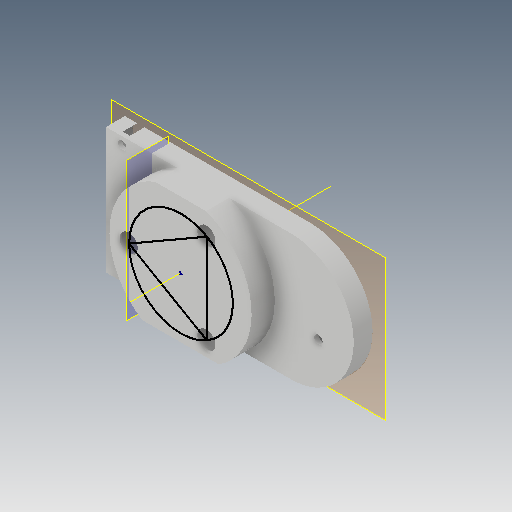
# Autodesk Inventor part: 03_Insert_Chip_solid
Saved by Autodesk Inventor 2019 (Build 230136000, 136)
## iProperties
Created: 2019-06-11
Part Number: 03_Insert_Chip_solid
Material: Generic
Document SubType Name: Modeling
Designer: diederichbenedict
Density: 1 g/cm^3
Appearance: Default
Author: diederichbenedict
Autodesk Inventor part; units mm, degrees
ref_plane "YZ Plane" through (0, 0, 0) normal (1, 0, 0) x (0, 1, 0)
ref_plane "XZ Plane" through (0, 0, 0) normal (0, 1, 0) x (-1, 0, 0)
ref_plane "XY Plane" through (0, 0, 0) normal (0, 0, 1) x (1, 0, 0)
ref_plane "Work Plane1" through (-1.2111, 0.775, 9.6) normal (0, 0, 1) x (0, -1, 0)
sketch "Sketch1" plane through (-1.2111, 0.775, 9.6) normal (0, 0, 1) x (0, -1, 0)
  circle A0 centre (3.575, 28.5389) radius 1.75 construction
  circle A1 centre (-13.125, -18.1803) radius 2 construction
  arc A2 (15.225, -15.8355) -> (15.225, -18.7868) centre (13.875, -17.3111) ccw construction
  line L0 (15.225, -15.8355) -> (15.225, 22.2111) construction
  arc A3 (15.225, 22.2111) -> (-15.225, 22.2111) centre (0, 21.8802) ccw construction
  line L1 (-15.225, 22.2111) -> (-15.225, -22.2111) construction
  line L2 (-15.225, -22.2111) -> (15.225, -22.2111) construction
  line L3 (15.225, -22.2111) -> (15.225, -18.7868) construction
  arc A4 (15.025, 22.209) -> (-15.025, 22.209) centre (0, 21.8802) ccw
  line L4 (15.025, 22.209) -> (15.025, -15.4356)
  arc A5 (15.025, -15.4356) -> (15.025, -19.1866) centre (13.875, -17.3111) ccw
  line L5 (15.025, -19.1866) -> (15.025, -22.0111)
  line L6 (15.025, -22.0111) -> (-14.956, -22.0111)
  arc A6 (-15.025, -18.8048) -> (-15.025, -17.5558) centre (-13.125, -18.1803) ccw construction
  circle A7 centre (3.575, 28.5389) radius 2.25
  arc A8 (-14.9598, -19.0514) -> (-14.9748, -17.3415) centre (-13.125, -18.1803) ccw
  line L7 (-14.956, -22.0111) -> (-14.9598, -19.0514)
  line L8 (-14.9748, -17.3415) -> (-15.025, 22.209)
  point P0 (0.775, 1.2111)
  dimension "d0" = 0.2
  dimension "d1" = 0.5
  constraints: 10 end point, 10 point on circle, 5 centre point, 1 coincident, 1 concentric, 1 parallel, 4 other
  measures "d0" radial gap between concentric circles of A3 A4
  measures "d1" radial gap between concentric circles of A0 A7
ref_plane "Work Plane2" through (21, -90, 18.7376) normal (0, 0, 1) x (1, 0, 0)
extrude "Extrusion1" add sketch "Sketch1" along normal blind 10
sketch "Sketch2" plane through (-16.6468, -14.25, 19.6) normal (0, 0, 1) x (1, 0, 0)
  circle A0 centre (16.6468, 14.25) radius 12.3406
  line L0 (4.3062, 14.25) -> (22.8171, 24.9373)
  line L1 (22.8171, 24.9373) -> (22.8171, 3.5627)
  line L2 (22.8171, 3.5627) -> (4.3062, 14.25)
  constraints: 6 end point, 2 coincident, 1 horizontal alignment, 9 other
ref_plane "Work Plane3" through (-12.3406, 0, 19.6) normal (-1, 0, 0) x (0, 0, 1)
sketch "Sketch3" plane through (-12.3406, 0, 19.6) normal (-1, 0, 0) x (0, 0, 1)
  line L0 (-0.8319, 0) -> (-10, 0)
  line L1 (-10, 15.8) -> (-10, -14.25) projected
  circle A0 centre (-1.4284, 0) radius 2.6
  line L2 (1.1716, 0) -> (-4.0284, 0)
  point P0 (-19.6, 0)
  dimension "d4" = 5.2
  constraints: 4 end point, 3 point on line, 2 point on circle, 1 centre point, 1 horizontal
  measures "d4" diameter of A0
revolve "Revolution1" cut sketch "Sketch3" angle 360 about axis through (-12.3406, 0, 18.7681) along (0, 0, -1) picked at (-2.9377, -0.2074) contours L2 A0 L0
pattern_circular "Circular Pattern1" count 3 over 360 about axis through (0, 0, 19.6) along (0, 0, 1) of "Revolution1"
ref_plane "Work Plane4" through (25.5777, -4.55, 13.1) normal (0, 0, 1) x (1, 0, 0)
sketch "Sketch5" plane through (-1.2111, 0.775, 19.6) normal (0, 0, 1) x (1, 0, 0)
  circle A0 centre (1.2111, -0.775) radius 16.9061
  circle A1 centre (7.3815, 9.9123) radius 2.1725 projected
  circle A2 centre (7.3815, -11.4623) radius 2.1725 projected
  circle A3 centre (-11.1295, -0.775) radius 2.1725 projected
  circle A4 centre (28.5389, -3.575) radius 2.25 projected
  arc A5 (22.209, -15.025) -> (22.209, 15.025) centre (21.8802, 0) ccw projected
  line L0 (22.209, 15.025) -> (-17.3415, 14.9748) projected
  arc A6 (-19.0514, 14.9598) -> (-17.3415, 14.9748) centre (-18.1803, 13.125) ccw projected
  line L1 (-19.0514, 14.9598) -> (-22.0111, 14.956) projected
  line L2 (-22.0111, 14.956) -> (-22.0111, -15.025) projected
  line L3 (-22.0111, -15.025) -> (-19.1866, -15.025) projected
  arc A7 (-15.4356, -15.025) -> (-19.1866, -15.025) centre (-17.3111, -13.875) ccw projected
  line L4 (-15.4356, -15.025) -> (22.209, -15.025) projected
  line L5 (22.209, 15.025) -> (-17.3415, 14.9748) projected
  line L6 (-15.4356, -15.025) -> (22.209, -15.025) projected
  point P0 (7.2754, 15.006)
  point P1 (-4.8932, 14.9906)
  point P2 (-7.8858, -15.025)
  point P3 (10.3081, -15.025)
  constraints: 4 point on circle, 4 point on line, 1 centre point, 1 coincident
extrude "Extrusion3" cut sketch "Sketch5" against normal up to surface (6.5 mm away) contours A0 L0 A5 L4 | A0 L4 A7 L3 L2 L1 A6 L0
sketch "Sketch6" plane through (-1.2111, 0.775, 13.1) normal (0, 0, 1) x (1, 0, 0)
  circle A0 centre (28.5389, -3.575) radius 2.25 projected
  arc A1 (22.209, -15.025) -> (22.209, 15.025) centre (21.8802, 0) ccw projected
  line L0 (7.2754, 15.006) -> (22.209, 15.025) projected
  arc A2 (10.3081, -15.025) -> (7.2754, 15.006) centre (1.2111, -0.775) ccw projected
  line L1 (22.209, -15.025) -> (10.3081, -15.025) projected
  arc A3 (-19.0514, 14.9598) -> (-17.3415, 14.9748) centre (-18.1803, 13.125) ccw projected
  line L2 (-22.0111, 14.956) -> (-19.0514, 14.9598) projected
  line L3 (-22.0111, -15.025) -> (-22.0111, 14.956) projected
  line L4 (-19.1866, -15.025) -> (-22.0111, -15.025) projected
  arc A4 (-15.4356, -15.025) -> (-19.1866, -15.025) centre (-17.3111, -13.875) ccw projected
  line L5 (-7.8858, -15.025) -> (-15.4356, -15.025) projected
  arc A5 (-4.8932, 14.9906) -> (-7.8858, -15.025) centre (1.2111, -0.775) ccw projected
  line L6 (-17.3415, 14.9748) -> (-4.8932, 14.9906) projected
  circle A6 centre (-18.1803, 13.125) radius 1
  circle A7 centre (-17.3111, -13.875) radius 1
  circle A8 centre (28.5389, -3.575) radius 1
  arc A9 (-19.0514, 14.9598) -> (-17.3415, 14.9748) centre (-18.1803, 13.125) ccw projected
  line L7 (-17.3415, 14.9748) -> (-19.0514, 14.9598)
  line L8 (-15.4356, -15.025) -> (-19.1866, -15.025)
  point P0 (1.2111, -0.775)
  dimension "d13" = 2
  dimension "d14" = 2
  dimension "d15" = 2
  constraints: 4 end point, 3 centre point, 3 coincident, 1 collinear
  measures "d13" diameter of A6
  measures "d14" diameter of A7
  measures "d15" diameter of A8
extrude "Extrusion4" add sketch "Sketch6" along normal blind 1 contours A0 | L1 A2 L0 A1 | L7 A3 | A3 L6 A5 L5 A4 L4 L3 L2 | A4 L8
body "Solid1"
